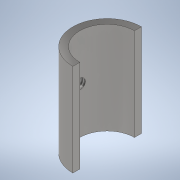
# Autodesk Inventor part: Half Pipe A53 - DN25-H45
Saved by Autodesk Inventor 2020.3 (Build 243373000, 373)
## iProperties
Created: 2020-06-30
Part Number: Half Pipe A53 - DN25-H45
Material: Steel, Carbon
Document SubType Name: Modeling
Designer: Bruno
Density: 7.85 g/cm^3
Appearance: Semi-Polished
Author: Bruno
Autodesk Inventor part; units mm, degrees
ref_plane "YZ Plane" through (0, 0, 0) normal (1, 0, 0) x (0, 1, 0)
ref_plane "XZ Plane" through (0, 0, 0) normal (0, 1, 0) x (-1, 0, 0)
sketch "Sketch1" plane through (0, 0, 0) normal (0, 1, 0) x (-1, 0, 0)
  arc A0 (0, -16.7) -> (0, 16.7) centre (0, 0) ccw
  arc A1 (0, -13.3) -> (0, 13.3) centre (0, 0) ccw
  line L0 (0, 16.7) -> (0, 13.3)
  line L1 (0, -13.3) -> (0, -16.7)
  dimension "d0" = 33.4
  dimension "d1" = 26.6
  constraints: 4 end point, 4 point on circle, 2 centre point, 2 coincident, 2 vertical
  measures "d0" diameter of A0
  measures "d1" diameter of A1
extrude "Extrusion1" add sketch "Sketch1" along normal blind 45
ref_plane "Work Plane1" through (-16.7, 0, 0) normal (1, 0, 0) x (0, 1, 0)
sketch "Sketch2" plane through (-16.7, 0, 0) normal (1, 0, 0) x (0, 1, 0)
  line L0 (45, -16.7) -> (45, 16.7) projected
  point P0 (0, 0)
  point P1 (22.5, 0)
  dimension "d4" = 22.5
  measures "d4" distance from line of L0 point (22.5, 0)
hole "Hole1" at (-16.7, 22.5, 0) direction (1, 0, 0) diameter 4.9784 end through all thread size "1/4-20 UNC" class "2B" standard "ANSI Unified Screw Threads"
body "Solid1"
